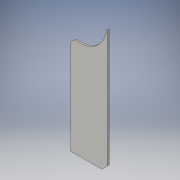
# Autodesk Inventor part: Backstopleft
Saved by Autodesk Inventor 2016 (Build 200138000, 138)
## iProperties
Created: 2017-01-16
Part Number: Backstopleft
Material: Generic
Document SubType Name: Modeling
Designer: RoboticsUser
Density: 1 g/cm^3
Appearance: Default
Author: RoboticsUser
Autodesk Inventor part; units mm, degrees
ref_plane "YZ Plane" through (0, 0, 0) normal (1, 0, 0) x (0, 1, 0)
ref_plane "XZ Plane" through (0, 0, 0) normal (0, 1, 0) x (-1, 0, 0)
ref_plane "XY Plane" through (0, 0, 0) normal (0, 0, 1) x (1, 0, 0)
sketch "Sketch1" plane through (0, 0, 0) normal (0, 0, 1) x (1, 0, 0)
  line L0 (0, 0) -> (82.55, 0)
  line L1 (82.55, 0) -> (82.55, 304.8)
  line L2 (82.55, 304.8) -> (0, 304.8)
  line L3 (0, 304.8) -> (0, 0)
  dimension "d0" = 82.55
  dimension "d1" = 304.8
  constraints: 8 end point, 2 parallel, 1 horizontal, 1 perpendicular
  measures "d0" distance of L2.end L1.end
  measures "d1" distance of L1.end L0.end
extrude "Extrusion1" add sketch "Sketch1" along normal blind 3.81
chamfer "Chamfer1" distance 12.7 angle 45 1 edges at (82.55, 0, 1.905)
hole "Hole1" at (17.78, 284.48, 3.81) direction (0, 0, -1) diameter 127 end through all
hole "Hole2" at (80.6545, 302.7787, 3.81) direction (0, 0, -1) diameter 48.26 end through all
fillet "Fillet1" radius 7.62 1 edges at (81.0119, 278.6513, 1.905)
fillet "Fillet2" radius 12.7 1 edges at (0, 223.52, 1.905)
body "Solid1"
